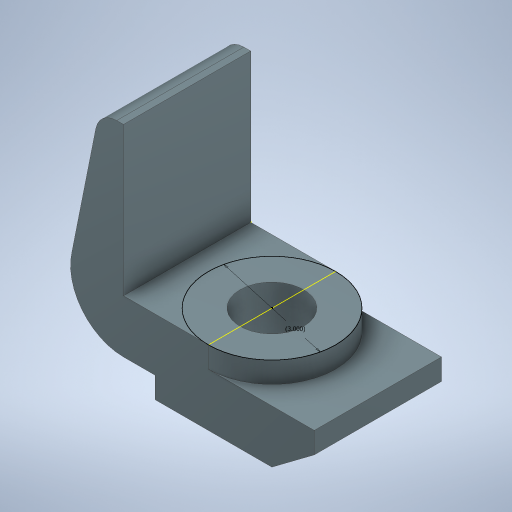
# Autodesk Inventor part: ASN4-3-BK
Saved by Autodesk Inventor 2024 (Build 280153000, 153)
## iProperties
Created: 2023-09-23
Part Number: ASN4-3-BK
Material: Brass, Soft Yellow
Document SubType Name: Modeling
Designer: bennk
Density: 8.47 g/cm^3
Appearance: White
Author: bennk
Autodesk Inventor part; units mm, degrees
ref_plane "YZ Plane" through (0, 0, 0) normal (1, 0, 0) x (0, 1, 0)
ref_plane "XZ Plane" through (0, 0, 0) normal (0, 1, 0) x (-1, 0, 0)
ref_plane "XY Plane" through (0, 0, 0) normal (0, 0, 1) x (1, 0, 0)
sketch "main profile" plane through (0, 0, 0) normal (0, 0, 1) x (1, 0, 0)
  line L0 (0, 0) -> (50.8, 0)
  line L1 (50.8, 0) -> (50.8, -12.7)
  line L2 (19.05, -31.75) -> (19.05, -44.45)
  line L3 (19.05, -44.45) -> (88.9, -44.45)
  line L4 (0, 0) -> (0, 76.1994)
  line L5 (50.8, -12.7) -> (114.3, -12.7)
  line L6 (114.3, -12.7) -> (114.3, -25.4)
  line L7 (88.9, -44.45) -> (114.3, -25.4)
  line L8 (0, 88.9) -> (-4.1016, 88.9)
  arc A0 (-4.1016, 88.9) -> (-16.5527, 78.7018) centre (-4.1016, 76.2) ccw
  line L9 (-16.5527, 78.7018) -> (-30.8986, 7.3033)
  arc A1 (-30.8986, 7.3033) -> (0, -31.75) centre (0, 0) ccw
  line L10 (19.05, -31.75) -> (0, -31.75)
  line L11 (0, 76.1994) -> (0, 88.9)
  point P0 (-6.35, 76.2)
  point P1 (-6.35, 76.2)
  point P2 (-6.35, 88.9)
  dimension "d8" = 50.8
  dimension "d9" = 12.7
  dimension "d11" = 69.85
  dimension "d15" = 114.3
  dimension "d16" = 12.7
  dimension "d18" = 44.45
  dimension "d20" = 19.05
  dimension "d39" = 6.35
  dimension "d41" = 12.7
  dimension "d42" = 31.75
  dimension "d44" = 31.75
  dimension "d45" = 120.65
  constraints: 24 end point, 5 point on circle, 4 perpendicular, 4 vertical, 2 centre point, 2 coincident, 2 horizontal, 2 tangent, 1 point on line
  measures "d8" distance of L0.start L0.end
  measures "d9" distance of L0.end L1.end
  measures "d11" distance of L2.end L3.end
  measures "d15" distance between parallel lines of L6 L4
  measures "d16" distance of L5.end L6.end
  measures "d18" distance between parallel lines of L3 L0
  measures "d20" distance between parallel lines of L2 L4
  measures "d39" distance of L8.start point (-6.35, 88.9)
  measures "d41" radius of A0
  measures "d42" radius of A1
  measures "d44" distance between parallel lines of L10 L0
  measures "d45" distance from line of L8.start L10
extrude "FULL EXTRUSION" add sketch "main profile" along normal blind 76.2
sketch "Half Circle" plane through (0, 0, 0) normal (0, 1, 0) x (1, 0, 0)
  line L0 (50.8, 0) -> (50.8, -76.2) projected
  circle A0 centre (50.8, -38.1) radius 38.1
  point P0 (0, 0)
  dimension "d55" = 76.2
  constraints: 1 midpoint, 1 vertical alignment, 2 other
extrude "Half Circle Extrusion" add sketch "Half Circle" against normal up to surface (12.7 mm away)
sketch "Sketch6" plane through (0, 0, 76.2) normal (0, 1, 0) x (1, 0, 0)
  arc A0 (50.8, 0) -> (50.8, 76.2) centre (50.8, 38.1) ccw projected
  point P0 (0, 76.2)
  constraints: 1 coincident
hole "Hole2" at (50.8, 0, 38.1) direction (0, -1, 0) diameter 38.1 end through all
equation "\"d16\" = d9"
body "Solid1"
